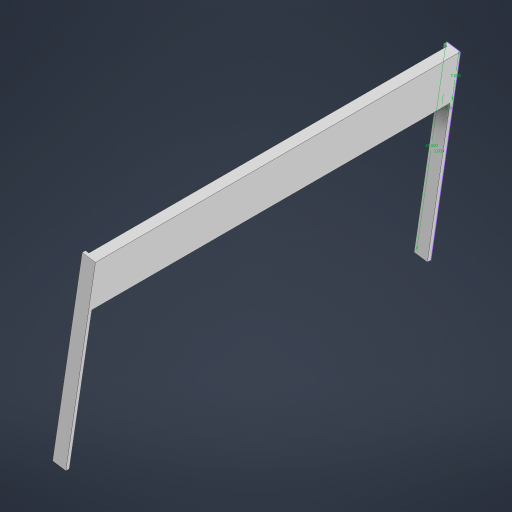
# Autodesk Inventor part: BackRest
Saved by Autodesk Inventor 2023 (Build 270158000, 158)
## iProperties
Created: 2026-02-03
Part Number: BackRest
Material: Generic
Document SubType Name: Modeling
Designer: ansle
Density: 1 g/cm^3
Appearance: Default
Author: ansle
Autodesk Inventor part; units mm, degrees
ref_plane "YZ Plane" through (0, 0, 0) normal (1, 0, 0) x (0, 1, 0)
ref_plane "XZ Plane" through (0, 0, 0) normal (0, 1, 0) x (-1, 0, 0)
ref_plane "XY Plane" through (0, 0, 0) normal (0, 0, 1) x (1, 0, 0)
sketch "Sketch1" plane through (0, 0, 0) normal (0, 0, 1) x (1, 0, 0)
  line L0 (0, 0) -> (112.2718, 740.8411)
  line L1 (50.2265, -7.6116) -> (162.4983, 733.2294)
  line L2 (162.4983, 733.2294) -> (112.2718, 740.8411)
  line L3 (50.2265, -7.6116) -> (0, 0)
  line L4 (162.4983, 733.2294) -> (135.8576, 557.4366)
  line L5 (135.8576, 557.4366) -> (98.1877, 563.1454)
  line L6 (98.1877, 563.1454) -> (124.8285, 738.9382)
  line L7 (124.8285, 738.9382) -> (162.4983, 733.2294)
  dimension "d0" = 749.3
  dimension "d2" = 50.8
  dimension "d3" = 177.8
  dimension "d4" = 38.1
  constraints: 16 end point, 3 perpendicular, 2 parallel, 2 point on line
  measures "d0" distance of L0.start L0.end
  measures "d2" distance between parallel lines of L0 L1
  measures "d3" distance of L1.end L4.end
  measures "d4" distance of L4.end L5.end
extrude "Extrusion1" add sketch "Sketch1" along normal blind 1384.3 contours L2 L1 L5 L6
extrude "Extrusion2" add sketch "Sketch1" along normal blind 12.7 contours L0 L2 L6 L5 L1 L3
sketch "Sketch2" plane through (0, 0, 1384.3) normal (0, 0, 1) x (1, 0, 0)
  line L0 (162.4983, 733.2294) -> (124.8285, 738.9382) projected
  line L1 (162.4983, 733.2294) -> (112.2718, 740.8411)
  line L2 (0, 0) -> (50.2265, -7.6116) projected
  line L3 (112.2718, 740.8411) -> (0, 0)
  line L4 (50.2265, -7.6116) -> (162.4983, 733.2294) projected
  line L5 (0, 0) -> (50.2265, -7.6116)
  line L6 (50.2265, -7.6116) -> (162.4983, 733.2294)
  line L7 (135.8576, 557.4366) -> (162.4983, 733.2294) projected
  line L8 (112.2718, 740.8411) -> (162.4983, 733.2294)
  line L9 (162.4983, 733.2294) -> (50.2265, -7.6116)
  dimension "d9" = 50.8
  constraints: 12 end point, 2 perpendicular, 1 collinear
  measures "d9" distance of L0.start L1.end
extrude "Extrusion3" add sketch "Sketch2" against normal blind 12.7
body "Solid1"
